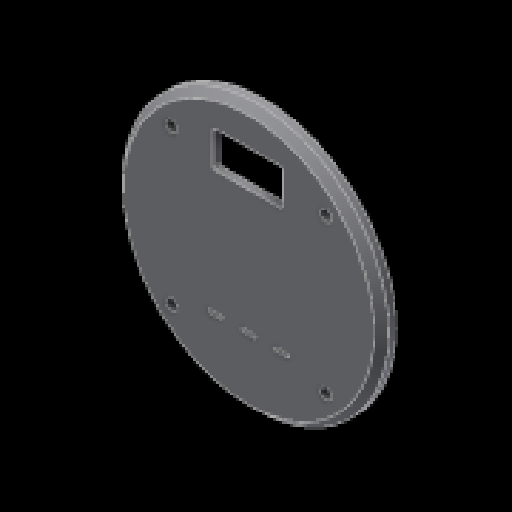
# Autodesk Inventor part: WheelEncoderCover
Saved by Autodesk Inventor 2025.2 (Build 292293000, 293)
## iProperties
Created: 2026-02-04
Part Number: WheelEncoderCover
Material: Generic
Document SubType Name: Modeling
Designer: valer
Density: 1 g/cm^3
Appearance: Default
Author: valer
Autodesk Inventor part; units mm, degrees
ref_plane "YZ Plane" through (0, 0, 0) normal (1, 0, 0) x (0, 1, 0)
ref_plane "XZ Plane" through (0, 0, 0) normal (0, 1, 0) x (-1, 0, 0)
ref_plane "XY Plane" through (0, 0, 0) normal (0, 0, 1) x (1, 0, 0)
sketch "Base" plane through (0, 0, 0) normal (0, 0, 1) x (1, 0, 0)
  circle A0 centre (0, 0) radius 36.125
  circle A1 centre (0, 0) radius 33.125
  circle A2 centre (0, 0) radius 34.625 construction
  dimension "d1" = 66.25
  dimension "d2" = 3
  dimension "d3" = 1.5
  constraints: 3 centre point, 3 coincident
  measures "d1" diameter of A1
  measures "d2" radial gap between concentric circles of A0 A1
  measures "d3" radial gap between concentric circles of A0 A2
extrude "BaseFeature" add sketch "Base" along normal blind 2
sketch "Cap" plane through (0, 0, 2) normal (0, 0, 1) x (1, 0, 0)
  circle A0 centre (0, 0) radius 36.125 projected
extrude "CapFeature" add sketch "Cap" along normal blind 2
chamfer "CapChamferFeature" distance 2 angle 45 1 edges at (-36.125, 0, 4)
sketch "MountHoles" plane through (0, 0, 4) normal (0, 0, 1) x (1, 0, 0)
  circle A0 centre (-20.9919, -21) radius 1.25 projected
  circle A1 centre (-20.9919, 21) radius 1.25 projected
  circle A2 centre (21.0081, -21) radius 1.25 projected
  circle A3 centre (21.0081, 21) radius 1.25 projected
hole "MountHolesFeature" at (-20.9919, -21, 4) at (-20.9919, 21, 4) at (21.0081, 21, 4) at (21.0081, -21, 4) direction (0, 0, -1) diameter 3 end through all
sketch "CapHoles" plane through (0, 0, 4) normal (0, 0, 1) x (1, 0, 0)
  line L0 (-7.125, -17.7082) -> (-11.125, -17.7082) projected
  line L1 (-11.125, -17.7082) -> (-11.125, -16.7082) projected
  line L2 (-7.125, -16.7082) -> (-7.125, -17.7082) projected
  line L3 (-11.125, -16.7082) -> (-7.125, -16.7082) projected
  line L4 (-2, -17.7082) -> (-2, -16.7082) projected
  line L5 (2, -17.7082) -> (-2, -17.7082) projected
  line L6 (-2, -16.7082) -> (2, -16.7082) projected
  line L7 (2, -16.7082) -> (2, -17.7082) projected
  line L8 (7.125, -17.7082) -> (7.125, -16.7082) projected
  line L9 (11.125, -17.7082) -> (7.125, -17.7082) projected
  line L10 (7.125, -16.7082) -> (11.125, -16.7082) projected
  line L11 (11.125, -16.7082) -> (11.125, -17.7082) projected
  line L12 (-9.125, 25.943) -> (-9.125, 17.093) construction
  line L13 (8.695, 17.093) -> (8.695, 25.943) construction
  line L14 (-9.125, 25.943) -> (8.695, 25.943) construction
  line L15 (-9.125, 17.093) -> (8.695, 17.093) construction
  line L16 (-9.625, 16.593) -> (-9.625, 26.443)
  line L17 (-9.625, 26.443) -> (9.195, 26.443)
  line L18 (9.195, 26.443) -> (9.195, 16.593)
  line L19 (9.195, 16.593) -> (-9.625, 16.593)
  point P0 (0, 0)
  dimension "d22" = 0.5
  constraints: 12 end point, 2 parallel, 1 horizontal, 3 other
  measures "d22" distance between parallel lines of L12 L16
extrude "CapHolesFeature" cut sketch "CapHoles" against normal through all
fillet "CapHoleFilletsFeature" radius 0.5 16 edges at (-9.625, 26.443, 3) (-9.625, 16.593, 3) (9.195, 26.443, 3) (9.195, 16.593, 3) (-11.125, -16.7082, 3) (-11.125, -17.7082, 3) (-7.125, -16.7082, 3) (-7.125, -17.7082, 3) (-2, -17.7082, 3) (-2, -16.7082, 3) (2, -17.7082, 3) (2, -16.7082, 3) (7.125, -17.7082, 3) (7.125, -16.7082, 3) (11.125, -17.7082, 3) (11.125, -16.7082, 3)
equation "\"d3\" = 0.5 * d2"
body "Solid1"
